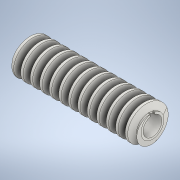
# Autodesk Inventor part: Worm
Saved by Autodesk Inventor 2020.3 (Build 243373000, 373)
## iProperties
CustomPartVersion: 1
Created: 2020-05-26
Part Number: Worm
Material: Steel, Mild
Document SubType Name: Modeling
Designer: robst
Categories: <?xml version="1.0" encoding="UTF-16"?> <MemberInstance><Categories><FamilyTemplate><FamilyTemplateParameter ValueType="xs:double" Id="1" ObjectReferenceKey="da_z" ObjectType="kUserParameterObject"/><FamilyTemplateParameter ValueType="xs:double" Id="2" ObjectReferenceKey="da_b" ObjectType="kUserParameterObject"/><FamilyTemplateParameter ValueType="xs:double" Id="3" ObjectReferenceKey="da_beta" ObjectType="kUserParameterObject"/><FamilyTemplateParameter ValueType="xs:double" Id="4" ObjectReferenceKey="da_m" ObjectType="kUserParameterObject"/><FamilyTemplateParameter ValueType="xs:double" Id="5" ObjectReferenceKey="da_alpha" ObjectType="kUserParameterObject"/><FamilyTemplateParameter ValueType="xs:double" Id="6" ObjectReferenceKey="da_da" ObjectType="kUserParameterObject"/><FamilyTemplateParameter ValueType="xs:double" Id="7" ObjectReferenceKey="da_aw" ObjectType="kUserParameterObject"/><FamilyTemplateParameter ValueType="xs:double" Id="8" ObjectReferenceKey="da_px" ObjectType="kUserParameterObject"/><FamilyTemplateParameter ValueType="xs:double" Id="9" ObjectReferenceKey="da_d" ObjectType="kUserParameterObject"/><FamilyTemplateParameter ValueType="xs:string" Id="10" ObjectReferenceKey="EAIAABAAAAC+GAAAAAAAAIAAAAAAAAAA" ObjectType="83910656" SubObjectId="SurfaceGeometry"/></FamilyTemplate><ParamToTemplateMap><ParamToTemplate CategoryParameter="//CategoryParameter[@InternalName='046C89C9-8512-4d59-83FE-43B91F4F132A']" TemplateParameter="1"/><ParamToTemplate CategoryParameter="//CategoryParameter[@InternalName='2552DF32-E462-4b46-AEBF-C6C7768E72AC']" TemplateParameter="2"/><ParamToTemplate CategoryParameter="//CategoryParameter[@InternalName='C9EE641D-15FC-4fae-A226-E94C4372FDD7']" TemplateParameter="3"/><ParamToTemplate><ParamToTemplate CategoryParameter="//CategoryParameter[@InternalName='00B6519A-459B-49c7-AD84-2E56D39A5744']" ConstantValue="0.000000"/></ParamToTemplate><ParamToTemplate><ParamToTemplate CategoryParameter="//CategoryParameter[@InternalName='04B31F0E-C7A6-4894-AA32-9629BEFACF47']" ConstantValue="1.000000"/></ParamToTemplate><ParamToTemplate><ParamToTemplate CategoryParameter="//CategoryParameter[@InternalName='43CBEC2E-7847-49e7-A936-2F7889FCB2D9']" ConstantValue="0.200000"/></ParamToTemplate><ParamToTemplate><ParamToTemplate CategoryParameter="//CategoryParameter[@InternalName='B1EFC894-105D-4ebd-86BF-FA20ED196853']" ConstantValue="0.266800"/></ParamToTemplate><ParamToTemplate><ParamToTemplate CategoryParameter="//CategoryParameter[@InternalName='51175063-3D10-4879-93E8-6246FE8B403D']" ConstantValue="2068427187.950509"/></ParamToTemplate><ParamToTemplate><ParamToTemplate CategoryParameter="//CategoryParameter[@InternalName='A3A52E27-4454-46a9-B0BD-C932399B70AF']" ConstantValue="0.270000"/></ParamToTemplate><ParamToTemplate CategoryParameter="//CategoryParameter[@InternalName='91B76062-C214-41d9-B1B9-14D2AB99603D']" TemplateParameter="4"/><ParamToTemplate CategoryParameter="//CategoryParameter[@InternalName='2D373A89-B862-43d6-8D0B-0CBF12AB9F6C']" TemplateParameter="5"/><ParamToTemplate CategoryParameter="//CategoryParameter[@InternalName='37777632-D6A2-4fac-9D53-DB8ACD95C989']" TemplateParameter="6"/><ParamToTemplate CategoryParameter="//CategoryParameter[@InternalName='FD1017F1-B727-4f7e-9707-0F86F1FF9423']" TemplateParameter="7"/><ParamToTemplate CategoryParameter="//CategoryParameter[@InternalName='3BF567DA-17EF-48d8-80EA-D119B07F6463']" TemplateParameter="8"/><ParamToTemplate CategoryParameter="//CategoryParameter[@InternalName='BF5A1E7E-5373-4a22-AAD3-F583781FCF3C']" TemplateParameter="9"/><ParamToTemplate><ParamToTemplate CategoryParameter="//CategoryParameter[@InternalName='D4F72237-D604-435a-AD0B-F738B7463A00']" ConstantValue="1.000000"/></ParamToTemplate><ParamToTemplate CategoryParameter="//CategoryParameter[@InternalName='27C3BAF2-7550-4e4b-AE2C-0DB134B7D9B7']" TemplateParameter="10"/></ParamToTemplateMap><Category DisplayName="Gear" InternalName="DC85795E-93AB-48d5-8EEE-5A27447B64BD" Mnemonic="Gear"><CategoryParameter DisplayName="z" InternalName="046C89C9-8512-4d59-83FE-43B91F4F132A" Mnemonic="z"/><CategoryParameter DisplayName="b|.1|" InternalName="2552DF32-E462-4b46-AEBF-C6C7768E72AC" Mnemonic="b"/><CategoryParameter DisplayName="||g|" InternalName="C9EE641D-15FC-4fae-A226-E94C4372FDD7" Mnemonic="beta"/><CategoryParameter DisplayName="x" InternalName="00B6519A-459B-49c7-AD84-2E56D39A5744" Mnemonic="x"/><CategoryParameter DisplayName="a*" InternalName="04B31F0E-C7A6-4894-AA32-9629BEFACF47" Mnemonic="a"/><CategoryParameter DisplayName="c*" InternalName="43CBEC2E-7847-49e7-A936-2F7889FCB2D9" Mnemonic="c"/><CategoryParameter DisplayName="r|.f|*" InternalName="B1EFC894-105D-4ebd-86BF-FA20ED196853" Mnemonic="rf"/><CategoryParameter DisplayName="E" InternalName="51175063-3D10-4879-93E8-6246FE8B403D" Mnemonic="E"/><CategoryParameter DisplayName="||m|" InternalName="A3A52E27-4454-46a9-B0BD-C932399B70AF" Mnemonic="mi"/><Category DisplayName="WormGear" InternalName="1B25C7EF-093B-4025-B3D3-619CD2A4550C" Mnemonic="WormGear"><CategoryParameter DisplayName="m" InternalName="91B76062-C214-41d9-B1B9-14D2AB99603D" Mnemonic="m"/><CategoryParameter DisplayName="||a|" InternalName="2D373A89-B862-43d6-8D0B-0CBF12AB9F6C" Mnemonic="alpha"/><CategoryParameter DisplayName="d|.a|" InternalName="37777632-D6A2-4fac-9D53-DB8ACD95C989" Mnemonic="da"/><CategoryParameter DisplayName="a|.w|" InternalName="FD1017F1-B727-4f7e-9707-0F86F1FF9423" Mnemonic="aw"/><CategoryParameter DisplayName="p|.x|" InternalName="3BF567DA-17EF-48d8-80EA-D119B07F6463" Mnemonic="px"/><CategoryParameter DisplayName="d" InternalName="BF5A1E7E-5373-4a22-AAD3-F583781FCF3C" Mnemonic="d"/><CategoryParameter DisplayName="k|.mat|" InternalName="D4F72237-D604-435a-AD0B-F738B7463A00" Mnemonic="Coef"/><CategoryParameter DisplayName="PitchDiameter" InternalName="27C3BAF2-7550-4e4b-AE2C-0DB134B7D9B7" Mnemonic="IDS_PITCHDIAM"/></Category></Category></Categories></MemberInstance>
Density: 7.86 g/cm^3
Appearance: Steel
Author: robst
Autodesk Inventor part; units mm, degrees
ref_plane "YZ Plane" through (0, 0, 0) normal (1, 0, 0) x (0, 1, 0)
ref_plane "XZ Plane" through (0, 0, 0) normal (0, 1, 0) x (-1, 0, 0)
ref_plane "XY Plane" through (0, 0, 0) normal (0, 0, 1) x (1, 0, 0)
sketch "Base Body Sketch" plane through (0, 0, 0) normal (1, 0, 0) x (0, 1, 0)
  circle A0 centre (0, 0) radius 9.217
  dimension "d5" = 18.434
extrude "Base Body" add sketch "Base Body Sketch" along normal mid plane 63.5
sketch "Sketch5" plane through (-31.75, 0, 0) normal (-1, 0, 0) x (0, 0, 1)
  circle A0 centre (0, 0) radius 9.217 projected
  circle A1 centre (0, 0) radius 7.6808
  dimension "d57" = 15.3616
  constraints: 1 centre point, 1 coincident
  measures "d57" diameter of A1
surface extrude "Pitch Diameter" sketch "Sketch5" against normal through all shown no curves A1
chamfer "Chamfer1" distance 1.2301 distance2 3.3796 1 edges at (31.75, -9.217, 0) measured on face at (31.25, -9.217, 0)
chamfer "Chamfer2" distance 1.2301 distance2 3.3796 1 edges at (-31.75, -9.217, 0) measured on face at (-31.25, -9.217, 0)
sketch "Tooth Sketch" plane through (0, 0, 0) normal (0, 0, 1) x (1, 0, 0)
  line L0 (0, 11.0038) -> (0, 5.6574) projected
  line L1 (-37.9942, 9.3092) -> (-36.7306, 5.8374)
  line L2 (-35.6594, 5.8374) -> (-34.3958, 9.3092)
  line L3 (-37.2766, 0) -> (-31.7352, 0) projected
  line L4 (-37.9942, 9.3092) -> (-36.195, 9.3092)
  line L5 (-36.195, 9.3092) -> (-34.3958, 9.3092)
  line L6 (-36.7306, 5.8374) -> (-36.195, 5.8374)
  line L7 (-36.195, 5.8374) -> (-35.6594, 5.8374)
  line L8 (-36.195, 7.6808) -> (-34.9885, 7.6808) construction
  line L9 (-36.195, 9.3092) -> (-36.195, 5.8374) construction
  dimension "d24" = 110
  dimension "d25" = 36.195
  dimension "d26" = 1.2065
  dimension "d27" = 5.8374
  dimension "d28" = 7.6808
  dimension "d29" = 9.3092
  constraints: 16 end point, 3 equal length, 3 parallel, 2 collinear, 2 point on line
  measures "d24" angle of L6 L1
  measures "d25" distance from line of L0 L4.end
  measures "d26" distance of L8.start L8.end
  measures "d27" distance between parallel lines of L3 L6
  measures "d28" distance between parallel lines of L3 L8
  measures "d29" distance between parallel lines of L3 L4
coil "Left Tooth" sketch "Tooth Sketch" operation cut axis through (-10, 0, 0) along (1, 0, 0) pitch 4.826 turns 16 hand left
pattern_of_one "Left Tooth Pattern"
feature "Tooth" [suppressed]
pattern_circular "Tooth Pattern" [suppressed]
sketch "Sketch14" plane through (31.75, 0, 0) normal (1, 0, 0) x (0, 0, -1)
  arc A0 (-1.1906, 4.6113) -> (1.1906, 4.6113) centre (0, 0) ccw
  line L0 (0, 0) -> (0, 4.7625) construction
  line L1 (0, 5.8019) -> (1.1906, 5.8019)
  line L2 (1.1906, 5.8019) -> (1.1906, 4.6113)
  line L3 (0, 5.8019) -> (-1.1906, 5.8019)
  line L4 (-1.1906, 5.8019) -> (-1.1906, 4.6113)
  dimension "d135" = 9.525
  dimension "oneHalfKey" = 1.1906
  dimension "d137" = 1.1906
  constraints: 10 end point, 2 point on circle, 2 symmetric about line, 1 centre point, 1 coincident, 1 horizontal, 1 point on line, 1 vertical
  measures "d135" diameter of A0
  measures "oneHalfKey" distance of L1.start L1.end
  measures "d137" distance of L1.end L2.end
extrude "Extrusion4" cut sketch "Sketch14" against normal through all
equation "\"d6\" = da_b"
equation "\"d8\" = fd_cham1"
equation "\"d9\" = 0.5 * fd_cham2"
equation "\"d10\" = fd_cham1"
equation "\"d11\" = 0.5 * fd_cham2"
equation "\"d25\" = fd_dist"
equation "\"d26\" = 0.25 * da_px"
equation "\"d27\" = 0.5 * da_df"
equation "\"d28\" = 0.5 * da_d"
equation "\"d29\" = 0.505 * da_da"
equation "\"d62\" = fd_n"
equation "\"da_rightdir\" = 0"
equation "\"d32\" = fd_n"
equation "\"d5\" = da_da"
equation "\"d57\" = da_d"
equation "\"da_aw\" = 76.80818"
equation "\"da_b\" = 63.5"
equation "\"da_df\" = 11.67484"
equation "\"da_da\" = 18.43396"
equation "\"fd_cham2\" = da_da - da_df"
equation "\"fd_cham1\" = 0.181985 * fd_cham2"
equation "\"da_d\" = 15.36164"
equation "\"da_px\" = 4.826"
equation "\"da_alfat\" = 20deg"
equation "\"d54\" = da_aw"
equation "\"d77\" = da_aw"
equation "\"d123\" = 0.125 * Sketch12_Pitch"
equation "\"Sketch12_Pitch\" = 1.27"
equation "\"d125\" = 60deg"
equation "\"fd_dist\" = 36.195"
equation "\"fd_n\" = 16"
body "Solid1"
body "Srf1"
